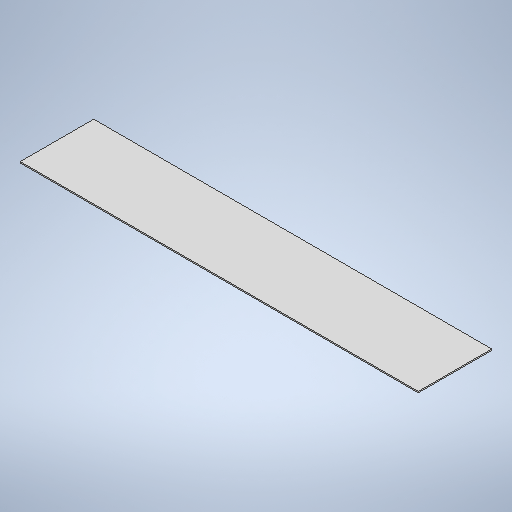
# Autodesk Inventor part: 025 TRM left board damper
Saved by Autodesk Inventor 2025 (Build 290162010, 162A)
## iProperties
Created: 2024-08-07
Part Number: 025 TRM left board damper
Material: AISI 304
Document SubType Name: Sheet Metal
Designer: pokla
Density: 8.02768 g/cm^3
Flat Pattern Width: 65 cm
Flat Pattern Length: 12 cm
Flat Pattern Area: 780 cm^2
Sheet Metal Rule: AISI304 2mm Die16
Sheet Metal Width: 650,000 mm
Sheet Metal Length: 120,000 mm
Sheet Metal Area: 78000,000 mm^2
Appearance: Default
Author: pokla
Autodesk Inventor part; units mm, degrees
ref_plane "YZ Plane" through (0, 0, 0) normal (1, 0, 0) x (0, 1, 0)
ref_plane "XZ Plane" through (0, 0, 0) normal (0, 1, 0) x (-1, 0, 0)
ref_plane "XY Plane" through (0, 0, 0) normal (0, 0, 1) x (1, 0, 0)
sketch "Sketch1" plane through (0, 0, 0) normal (0, 0, 1) x (1, 0, 0)
  line L0 (-325, -60) -> (325, -60)
  line L1 (325, -60) -> (325, 60)
  line L2 (325, 60) -> (-325, 60)
  line L3 (-325, 60) -> (-325, -60)
  line L4 (-325, -60) -> (325, 60) construction
  line L5 (325, -60) -> (-325, 60) construction
  point P0 (0, 0)
  dimension "d0" = 650
  dimension "d1" = 120
  measures "d0" distance of L2.end L1.end
  measures "d1" distance of L1.end L0.end
extrude "Plate1" add sketch "Sketch1" along normal blind 2
sketch "Sketch2" plane through (0, 0, 0) normal (0, 0, -1) x (-1, 0, 0)
  line L0 (-305, 40) -> (-105, 40) construction
  line L1 (-105, 40) -> (-105, 20) construction
  line L2 (-105, 20) -> (-305, 20) construction
  line L3 (-305, 20) -> (-305, 40) construction
  line L4 (-325, 60) -> (325, 60) projected
  line L5 (-325, -60) -> (-325, 60) projected
  point P0 (0, 0)
  point P1 (-48, 100)
  point P2 (325, 60)
  point P3 (-50, 98)
  dimension "d6" = 200
  dimension "d9" = 20
  dimension "d10" = 20
  dimension "d11" = 20
  constraints: 4 other
  measures "d6" distance of L0.start L0.end
  measures "d9" distance of L0.end L1.end
  measures "d11" length of L3
mark "Mark1"
equation "\"d2\" = Thickness"
equation "\"BendReliefWidth\" = Thickness"
equation "\"BendReliefDepth\" = 0.5 * Thickness"
equation "\"CornerReliefSize\" = 4 * Thickness"
equation "\"MinimumRemnant\" = 2 * Thickness"
equation "\"TransitionRadius\" = BendRadius"
equation "\"JacobiRadiusSize\" = BendRadius"
equation "\"GapSize\" = Thickness"
equation "\"Thickness\" = 2"
equation "\"BendRadius\" = 2.75"
body "Solid1"
